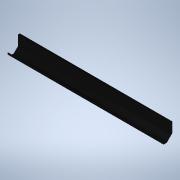
# Autodesk Inventor part: Rear_Rail_Wire_Cover
Saved by Autodesk Inventor 2022 (Build 260153000, 153)
## iProperties
Created: 2022-01-05
Part Number: Rear_Rail_Wire_Cover
Material: Generic
Document SubType Name: Modeling
Designer: derek
Density: 1 g/cm^3
Appearance: Glossy - Black
Author: derek
Autodesk Inventor part; units mm, degrees
ref_plane "YZ Plane" through (0, 0, 0) normal (1, 0, 0) x (0, 1, 0)
ref_plane "XZ Plane" through (0, 0, 0) normal (0, 1, 0) x (-1, 0, 0)
ref_plane "XY Plane" through (0, 0, 0) normal (0, 0, 1) x (1, 0, 0)
sketch "Sketch1" plane through (0, 0, 0) normal (1, 0, 0) x (0, 1, 0)
  line L0 (0, 0) -> (4, 0)
  line L1 (4, 0) -> (4, 20)
  line L2 (4, 20) -> (0, 20) construction
  line L3 (0, 20) -> (0, 0)
  line L4 (4, 20) -> (12, 28)
  line L5 (12, 28) -> (16, 28)
  line L6 (16, 28) -> (24, 20)
  line L7 (24, 20) -> (24, 24)
  line L8 (24, 24) -> (17.1716, 30.8284)
  line L9 (17.1716, 30.8284) -> (10.8284, 30.8284)
  line L10 (10.8284, 30.8284) -> (0, 20)
  line L11 (24, 20) -> (4, 20) construction
  line L12 (14, 30.8284) -> (14, 28) construction
  dimension "d0" = 20
  dimension "d1" = 4
  dimension "d8" = 135
  dimension "d11" = 20
  dimension "d12" = 8
  dimension "d13" = 2.8284
  dimension "d14" = 2.8284
  constraints: 26 end point, 6 perpendicular, 3 horizontal, 3 parallel, 2 midpoint
  measures "d0" distance of L2.end L0.start
  measures "d1" distance of L0.start L0.end
  measures "d8" angle of L5 L6
  measures "d11" distance between parallel lines of L1 L7
  measures "d12" distance between parallel lines of L11 L5
  measures "d13" distance between parallel lines of L5 L9
  measures "d14" distance between parallel lines of L6 L8
extrude "Extrusion1" add sketch "Sketch1" along normal blind 300
sketch "Sketch2" plane through (0, 0, 0) normal (0, -1, 0) x (1, 0, 0)
  line L0 (300, 0) -> (300, 20) projected
  line L1 (300, 10) -> (275, 10)
  line L2 (275, 10) -> (150, 10)
  line L3 (150, 10) -> (25, 10)
  line L4 (25, 10) -> (0, 10)
  line L5 (0, 0) -> (300, 0) projected
  line L6 (0, 20) -> (0, 0) projected
  dimension "d15" = 10
  dimension "d16" = 25
  constraints: 8 end point, 3 point on line, 2 collinear, 2 midpoint, 1 horizontal
  measures "d15" distance between parallel lines of L5 L4
  measures "d16" distance of L1.start L1.end
hole "Hole1" at (275, 0, 10) at (150, 0, 10) at (25, 0, 10) direction (0, 1, 0) diameter 3.4 end through all counterbore diameter 6.5 counterbore depth 1 clearance for "Socket Head Cap Screw" size "M3" standard "Ansi Metric M Profile"
move or copy body "Rotate1" bodies to move or copy 1 copy no rotation origin (0, 0, 0) rotation axis (1, 0, 0) rotation angle 90 translate (0, 14, 6)
equation "\"d13\" = d14"
body "Solid1"
